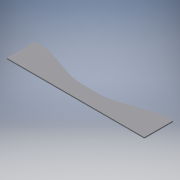
# Autodesk Inventor part: type7_base
Saved by Autodesk Inventor 2018.1 (Build 221171000, 171)
## iProperties
Created: 2017-11-03
Part Number: type7_base
Material: CFRP
Document SubType Name: Modeling
Designer: ku_sk
Density: 1.43 g/cm^3
Appearance: カーボンファイバー
Mass: 3609.32 g
Surface Area: 5347.72 cm^2
Volume: 2524 cm^3
Author: ku_sk
Autodesk Inventor part; units mm, degrees
ref_plane "YZ Plane" through (0, 0, 0) normal (1, 0, 0) x (0, 1, 0)
ref_plane "XZ Plane" through (0, 0, 0) normal (0, 1, 0) x (-1, 0, 0)
ref_plane "XY Plane" through (0, 0, 0) normal (0, 0, 1) x (1, 0, 0)
sketch "スケッチ1" plane through (0, 0, 0) normal (0, 1, 0) x (-1, 0, 0)
  line L0 (620, -125) -> (-620, -125)
  line L1 (-620, -125) -> (-620, 125)
  line L2 (-620, 125) -> (620, 125)
  line L3 (620, 125) -> (620, -125)
  line L4 (0, -175) -> (0, 175) projected
  line L5 (868, 0) -> (-868, 0) projected
  point P0 (0, 0)
  point P1 (0, -125)
  point P2 (620, 0)
  dimension "d0" = 1240
  dimension "d1" = 250
  constraints: 8 end point, 2 midpoint, 2 parallel, 2 point on line, 1 horizontal, 1 perpendicular
  measures "d0" distance of L0.start L0.end
  measures "d1" distance of L0.end L1.end
extrude "押し出し1" add sketch "スケッチ1" along normal blind 10
sketch "スケッチ2" plane through (0, 10, 0) normal (0, 1, 0) x (1, 0, 0)
  line L0 (0, 175) -> (0, -175) projected
  line L1 (0, 45) -> (200, 45)
  line L2 (200, 45) -> (520, 125)
  line L3 (620, 125) -> (-620, 125) projected
  line L4 (0, 45) -> (-200, 45)
  line L5 (-200, 45) -> (-520, 125)
  line L6 (620, -125) -> (620, 125) projected
  line L7 (-520, 125) -> (520, 125)
  line L8 (-620, -125) -> (620, -125) projected
  point P0 (0, 0)
  dimension "d5" = 200
  dimension "d6" = 100
  dimension "d10" = 170
  constraints: 10 end point, 2 point on line, 2 symmetric about line, 1 collinear, 1 horizontal
  measures "d5" distance of L1.start L1.end
  measures "d6" distance from line of L6 L2.end
  measures "d10" distance between parallel lines of L8 L1
extrude "押し出し2" cut sketch "スケッチ2" against normal through all contours L3 L2 L1 L0 | L0 L4 L5 L3
fillet "フィレット1" radius 500 4 edges at (-520, 5, -125) (-200, 5, -45) (200, 5, -45) (520, 5, -125)
